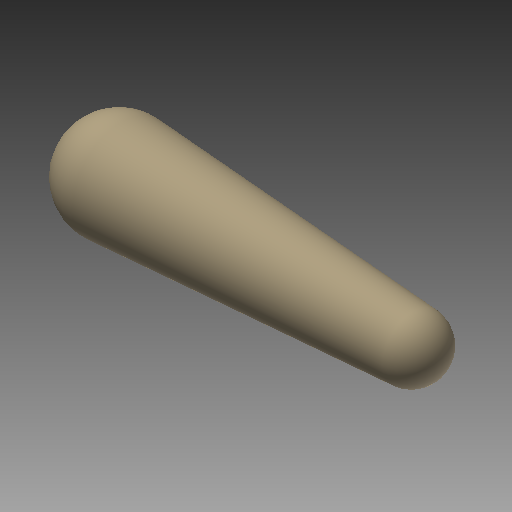
# Autodesk Inventor part: 3D HUMAN
Saved by Autodesk Inventor 2022 (Build 260153000, 153)
## iProperties
Category: PART
Part Number: 3D HUMAN
Document SubType Name: Modeling
Created: 2003-03-23
Designer: M.F.
Catalog Web Link: www.apollocanard.com
Density: 1 g/cm^3
Material: Generic
Appearance: Wheat
Control State: 0
Master: False
Checked Out: False
Shininess: 64.0
Length Units: 11272
Angle Units: 11279
Time Units: 11290
Mass Units: 11286
Length Display Precision: 3
Angle Display Precision: 2
Compacted: True
Density: 0.0
Volumn: 0.0
Area: 0.0
PropertySet Name: Model Information
Title: iMan
Author: M.F.
Autodesk Inventor part; units mm, degrees
ref_plane "YZ Plane" through (0, 0, 0) normal (1, 0, 0) x (0, 1, 0)
ref_plane "XZ Plane" through (0, 0, 0) normal (0, 1, 0) x (-1, 0, 0)
ref_plane "XY Plane" through (0, 0, 0) normal (0, 0, 1) x (1, 0, 0)
sketch "Sketch1" plane through (0, 0, 0) normal (0, 0, 1) x (1, 0, 0)
  circle A0 centre (0, 0) radius 44.069
  circle A1 centre (0, -260.096) radius 27.686
  line L0 (0, 44.069) -> (0, -287.782)
  line L1 (43.9815, -2.7758) -> (27.631, -261.8399)
  dimension "d16" = 260.096
  dimension "d17" = 88.138
  dimension "d18" = 55.372
  constraints: 4 end point, 4 point on circle, 2 centre point, 2 tangent, 1 coincident, 1 point on line, 1 vertical, 1 vertical alignment
  measures "d16" distance of A1.centre A0.centre
  measures "d17" diameter of A0
  measures "d18" diameter of A1
revolve "Revolution1" add sketch "Sketch1" angle 360 about axis through (0, 44.069, 0) along (0, -1, 0) picked at (10.3872, 10.3872) picked at (12.7574, -268.1195) contours A0 L0 | L1 A1 L0 A0 | A1 L0
equation "\"d16\" = ELBOW_TO_WRIST"
equation "\"d17\" = ELBOW_THK"
equation "\"d18\" = WRIST_THK"
equation "\"ELBOW_TO_WRIST\" = 260.096"
equation "\"ELBOW_THK\" = 88.138"
equation "\"WRIST_THK\" = 55.372"
body "Solid1"
